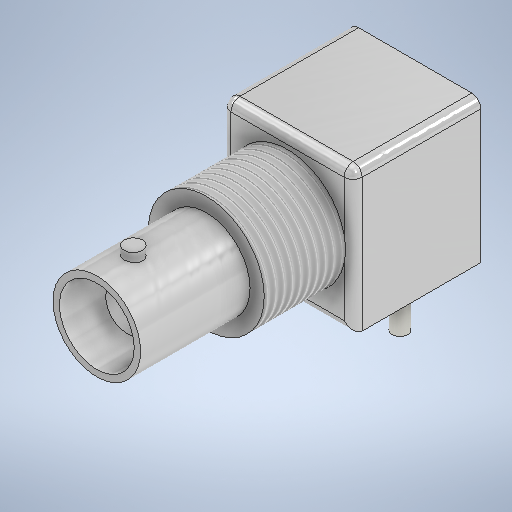
# Autodesk Inventor part: 031-5640
Saved by Autodesk Inventor 2025 (Build 290162000, 162)
## iProperties
Created: 2026-07-22
Part Number: 031-5640
Material: Generic
Document SubType Name: Modeling
Designer: Tapendra BC
Density: 1 g/cm^3
Appearance: Default
Catalog Web Link: https://www.digikey.ca/en/products/detail/amphenol-rf/031-5640/3593524
Description: CONN BNC JACK R/A 50 OHM PCB
Vendor: Digikey
Author: Tapendra BC
Comments: CONN BNC JACK R/A 50 OHM PCB
Revision Number: 1.0
Autodesk Inventor part; units mm, degrees
ref_plane "YZ Plane" through (0, 0, 0) normal (1, 0, 0) x (0, 1, 0)
sketch "Sketch5" plane through (0, 0, 0) normal (0, 0, 1) x (1, 0, 0)
  line L0 (-7.2, 7.8) -> (7.2, 7.8)
  line L1 (7.2, 7.8) -> (7.2, -7.8)
  line L2 (7.2, -7.8) -> (-7.2, -7.8)
  line L3 (-7.2, -7.8) -> (-7.2, 7.8)
  line L4 (-7.2, 7.8) -> (7.2, -7.8) construction
  line L5 (7.2, 7.8) -> (-7.2, -7.8) construction
  point P0 (0, 0)
  dimension "d7" = 14.4
  dimension "d8" = 15.6
  constraints: 12 end point, 2 midpoint, 2 parallel, 1 horizontal, 1 perpendicular
  measures "d7" distance of L0.start L0.end
  measures "d8" distance of L2.end L0.start
extrude "Extrusion3" add sketch "Sketch5" along normal blind 14
sketch "Sketch6" plane through (0, 0, 14) normal (0, 0, 1) x (1, 0, 0)
  circle A0 centre (0, 0) radius 6.35
  dimension "d11" = 12.7
  constraints: 1 centre point, 1 coincident
  measures "d11" diameter of A0
extrude "Extrusion4" add sketch "Sketch6" along normal blind 8.9
thread "Thread1"
fillet "Fillet1" radius 1 6 edges at (0, 7.8, 14) (7.2, 0, 14) (-7.2, 0, 14) (7.2, 7.8, 7) (-7.2, 7.8, 7) (0, -7.8, 14)
sketch "Sketch7" plane through (0, 0, 22.9) normal (0, 0, 1) x (1, 0, 0)
  circle A0 centre (0, 0) radius 4.8
  circle A1 centre (0, 0) radius 4.1
  dimension "d17" = 9.6
  dimension "d20" = 8.2
  constraints: 2 centre point, 2 coincident
  measures "d17" diameter of A0
  measures "d20" diameter of A1
extrude "Extrusion5" add sketch "Sketch7" along normal blind 12
ref_plane "Work Plane2" through (0, 0, 30.9) normal (0, 0, 1) x (1, 0, 0)
sketch "Sketch8" plane through (0, 0, 30.9) normal (0, 0, 1) x (1, 0, 0)
  circle A0 centre (0, 0) radius 4.8 projected
  line L0 (0, 4.8) -> (0, 5.7)
  line L1 (0, 5.7) -> (-1, 5.7)
  line L2 (-1, 4.6947) -> (-1, 5.7)
  arc A1 (0, 4.8) -> (-1, 4.6947) centre (0, 0) ccw
  circle A2 centre (0, 0) radius 4.1 projected
  line L3 (-4.1, 0) -> (4.1, 0) construction
  line L4 (0, -4.8) -> (0, -5.7)
  line L5 (0, -5.7) -> (-1, -5.7)
  line L6 (-1, -4.6947) -> (-1, -5.7)
  arc A3 (-1, -4.6947) -> (0, -4.8) centre (0, 0) ccw
  dimension "d22" = 0.9
  dimension "d23" = 1
  constraints: 14 end point, 8 point on circle, 4 symmetric about line, 2 centre point, 2 vertical, 1 concentric, 1 horizontal, 1 perpendicular, 1 other
  measures "d22" distance of L0.start L0.end
  measures "d23" distance of L0.end L1.end
revolve "Revolution1" add sketch "Sketch8" angle 360 about axis through (0, -4.8, 30.9) along (0, -1, 0) contours A0 L2 L1 L0 | L4 L5 L6 A0
sketch "Sketch9" plane through (0, 0, 22.9) normal (0, 0, 1) x (1, 0, 0)
  circle A0 centre (0, 0) radius 2.35
  circle A1 centre (0, 0) radius 0.3703
  dimension "d25" = 4.7
  constraints: 2 centre point, 2 coincident
  measures "d25" diameter of A0
extrude "Extrusion6" add sketch "Sketch9" along normal blind 8.68
sketch "Sketch10" plane through (-7.2, -7.8, 0) normal (0, -1, 0) x (1, 0, 0)
  circle A0 centre (12.28, 6.75) radius 0.865
  line L0 (13.4, 14) -> (1, 14) projected
  line L1 (7.2, 0) -> (7.2, 13) construction
  line L2 (0, 13) -> (14.4, 13) projected
  circle A1 centre (2.12, 6.75) radius 0.865
  dimension "d28" = 1.73
  dimension "d29" = 7.25
  dimension "d30" = 5.08
  constraints: 2 centre point, 2 end point, 1 midpoint, 1 symmetric about line, 1 other
  measures "d28" diameter of A0
  measures "d29" distance from line of L0 A0.centre
  measures "d30" distance from line of A0.centre L1
extrude "Extrusion7" add sketch "Sketch10" along normal blind 4.1
sketch "Sketch11" plane through (0, 0, 0) normal (0, 0, -1) x (-1, 0, 0)
  line L0 (-3.25, 6.4) -> (3.25, 6.4)
  line L1 (6.2, 6.8) -> (-6.2, 6.8) projected
  line L2 (-6.2, 7.8) -> (6.2, 7.8) projected
  line L3 (5.8, 3.3) -> (5.8, -3.3)
  line L4 (7.2, 6.8) -> (7.2, -7.8) projected
  line L5 (-5.8, 3.3) -> (-5.8, -3.3)
  line L6 (-7.2, -7.8) -> (-7.2, 6.8) projected
  line L7 (7.2, -7.8) -> (-7.2, -7.8) projected
  line L8 (-3.8, -7.8) -> (-3.8, -3.5)
  line L9 (3.9, -7.8) -> (3.9, -3.5)
  arc A0 (-5.8, 3.3) -> (-3.25, 6.4) centre (-5.4343, 5.598) ccw
  arc A1 (3.25, 6.4) -> (5.8, 3.3) centre (5.3258, 5.5087) ccw
  arc A2 (5.8, -3.3) -> (3.9, -3.5) centre (4.9374, -4.2303) ccw
  arc A3 (-3.8, -3.5) -> (-5.8, -3.3) centre (-4.8508, -3.9085) ccw
  line L10 (-3.8, -7.8) -> (3.9, -7.8)
  point P0 (0, 0)
  dimension "d33" = 1.4
  dimension "d34" = 1.4
  dimension "d35" = 1.4
  dimension "d36" = 3.4
  dimension "d37" = 3.3
  dimension "d38" = 4.3
  dimension "d39" = 4.3
  dimension "d40" = 6.6
  dimension "d41" = 6.6
  dimension "d42" = 6.5
  dimension "d43" = 3.95
  dimension "d44" = 4.5
  dimension "d45" = 4.5
  constraints: 12 end point, 8 point on circle, 4 centre point, 3 vertical, 2 point on line, 1 collinear, 1 parallel, 1 perpendicular
  measures "d33" distance between parallel lines of L2 L0
  measures "d34" distance between parallel lines of L4 L3
  measures "d35" distance between parallel lines of L6 L5
  measures "d36" distance between parallel lines of L8 L6
  measures "d37" distance between parallel lines of L4 L9
  measures "d38" distance of L9.start L9.end
  measures "d39" distance of L8.start L8.end
  measures "d40" distance of L3.start L3.end
  measures "d41" distance of L5.start L5.end
  measures "d42" distance of L0.start L0.end
  measures "d43" distance from line of L6 L0.start
  measures "d44" distance from line of L7 L5.end
  measures "d45" distance from line of L7 L3.end
extrude "Extrusion8" cut sketch "Sketch11" against normal blind 4.5
sketch "Sketch12" plane through (0, 0, 4.5) normal (0, 0, -1) x (-1, 0, 0)
  circle A0 centre (0, 0.25) radius 0.38
  line L0 (3.9, -7.8) -> (-3.8, -7.8) projected
  circle A1 centre (-2.54, 0.25) radius 0.36
  point P0 (0, 0)
  dimension "d48" = 8.05
  dimension "d49" = 0.76
  dimension "d50" = 0.72
  dimension "d51" = 2.54
  constraints: 2 centre point
  measures "d48" distance from line of A0.centre L0
  measures "d49" diameter of A0
  measures "d50" diameter of A1
  measures "d51" distance of A0.centre A1.centre
ref_plane "Work Plane3" through (0, 0.25, 4.5) normal (1, 0, 0) x (0, 0, -1)
sketch "Sketch14" plane through (0, 0.25, 4.5) normal (1, 0, 0) x (0, 0, -1)
  line L0 (0, 3.05) -> (0, -3.55) projected
  line L1 (0, 0) -> (1.33, 0)
  line L2 (2.83, -12.15) -> (2.83, -1.5)
  line L3 (-9.5, -7.05) -> (-9.5, -1.622) projected
  line L4 (4.5, -8.05) -> (-8.5, -8.05) projected
  arc A0 (2.83, -1.5) -> (1.33, 0) centre (1.33, -1.5) ccw
  point P0 (4.5, -0.25)
  dimension "d53" = 12.33
  dimension "d54" = 8.05
  dimension "d55" = 1.5
  constraints: 4 end point, 2 point on circle, 2 tangent, 1 centre point, 1 horizontal, 1 point on line, 1 vertical
  measures "d53" distance between parallel lines of L2 L3
  measures "d54" distance between parallel lines of L4 L1
  measures "d55" radius of A0
sweep "Sweep2" add profiles "Sketch12" path "Sketch14" path curves L1 A0 L2
equation "\"d34\" = d33"
equation "\"d35\" = d33"
equation "\"d39\" = d38"
equation "\"d41\" = d40"
equation "\"d45\" = d44"
body "Solid3"
